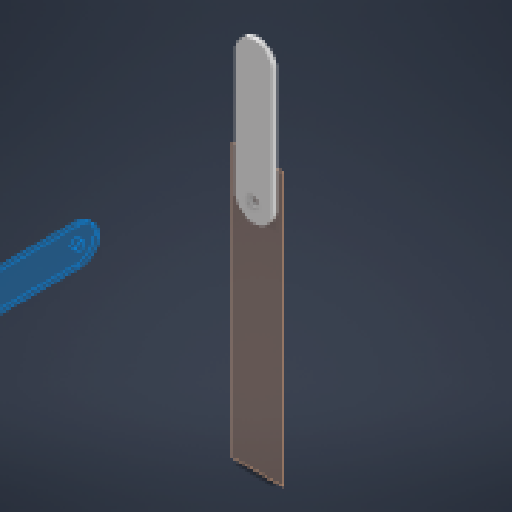
# Autodesk Inventor part: Link3base
Saved by Autodesk Inventor 2023 (Build 270158000, 158)
## iProperties
Created: 2023-09-09
Part Number: Link3base
Material: Generic
Document SubType Name: Modeling
Designer: philo
Density: 1 g/cm^3
Appearance: Default
Author: philo
Autodesk Inventor part; units mm, degrees
ref_plane "YZ Plane" through (0, 0, 0) normal (1, 0, 0) x (0, 1, 0)
ref_plane "XZ Plane" through (0, 0, 0) normal (0, 1, 0) x (-1, 0, 0)
ref_plane "XY Plane" through (0, 0, 0) normal (0, 0, 1) x (1, 0, 0)
ref_plane "Work Plane1" through (0, 0, 0) normal (0, 0, 1) x (1, 0, 0)
sketch "Sketch1" plane through (0, 0, 0) normal (0, 0, 1) x (1, 0, 0)
  circle A0 centre (0, 107.5) radius 10 projected
  circle A1 centre (0, 107.5) radius 5 projected
  line L0 (20, 237.5) -> (-20, 237.5)
  line L1 (-20, 237.5) -> (-20, 87.5)
  line L2 (-20, 87.5) -> (20, 87.5)
  line L3 (20, 87.5) -> (20, 237.5)
  circle A2 centre (0, 107.5) radius 20
  circle A3 centre (0, 237.5) radius 20
  point P0 (0, 0)
  point P1 (-20, 107.5)
  point P2 (20, 107.5)
  dimension "d0" = 40
  dimension "d1" = 150
  dimension "d2" = 20
  dimension "d4" = 20
  dimension "d5" = 40
  dimension "d6" = 130
  constraints: 8 end point, 2 centre point, 2 parallel, 1 coincident, 1 horizontal, 1 perpendicular
  measures "d0" distance of L2.end L1.end
  measures "d1" distance of L1.end L0.end
  measures "d2" distance from line of point (0, 0) L3
  measures "d4" distance from line of A0.centre L2
  measures "d5" diameter of A3
  measures "d6" distance of A3.centre A2.centre
extrude "Extrusion1" add sketch "Sketch1" along normal blind 5 contours A0 | A3 L0 | L0 A3 | L3 A2 L1 A3 | A2
body "Solid1"
